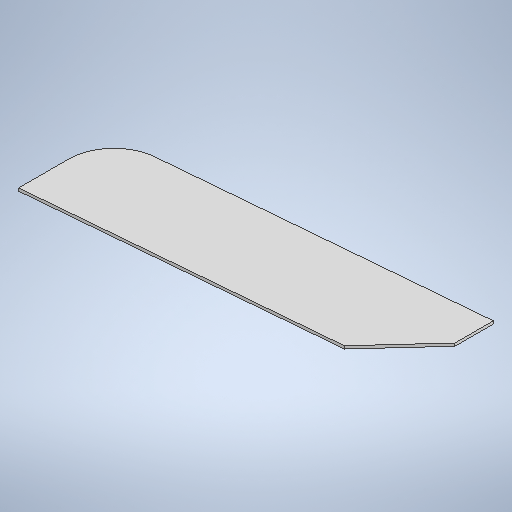
# Autodesk Inventor part: c
Saved by Autodesk Inventor 2025.2 (Build 292293000, 293)
## iProperties
Created: 2026-02-05
Part Number: c
Material: Generic
Document SubType Name: Modeling
Designer: Joefi
Density: 1 g/cm^3
Appearance: Default
Author: Joefi
Autodesk Inventor part; units mm, degrees
ref_plane "YZ Plane" through (0, 0, 0) normal (1, 0, 0) x (0, 1, 0)
ref_plane "XZ Plane" through (0, 0, 0) normal (0, 1, 0) x (-1, 0, 0)
ref_plane "XY Plane" through (0, 0, 0) normal (0, 0, 1) x (1, 0, 0)
sketch "Sketch1" plane through (0, 0, 0) normal (0, 1, 0) x (-1, 0, 0)
  line L0 (-55.6159, -9.9971) -> (-55.6159, -9.3981)
  arc A0 (-54.3022, -6.0201) -> (-55.6159, -9.3981) centre (-50.6159, -9.3981) ccw
  line L1 (-54.3022, -6.0201) -> (-42.899, 6.4243)
  arc A1 (-39.6484, 8.0273) -> (-42.899, 6.4243) centre (-39.2126, 3.0463) ccw
  line L2 (-39.6484, 8.0273) -> (35.5678, 14.6079)
  arc A2 (41.0036, 9.6269) -> (35.5678, 14.6079) centre (36.0036, 9.6269) ccw
  line L3 (41.0036, 9.6269) -> (41.0036, 3.0791)
  arc A3 (30.9623, -7.8791) -> (41.0036, 3.0791) centre (30.0036, 3.0791) ccw
  line L4 (30.9623, -7.8791) -> (-50.1801, -14.9781)
  arc A4 (-55.6159, -9.9971) -> (-50.1801, -14.9781) centre (-50.6159, -9.9971) ccw
  line L5 (-42.5345, 9.7825) -> (-57.6159, -6.6759)
  line L6 (-57.6159, -6.6759) -> (-57.6159, -17.6363)
  line L7 (-57.6159, -17.6363) -> (31.1366, -9.8715)
  arc A5 (31.1366, -9.8715) -> (43.0036, 3.0791) centre (30.0036, 3.0791) ccw
  line L8 (43.0036, 3.0791) -> (43.0036, 17.2661)
  line L9 (43.0036, 17.2661) -> (-42.5345, 9.7825)
  line L10 (-42.4396, 9.59) -> (-57.4159, -6.7537)
  line L11 (-57.4159, -6.7537) -> (-57.4159, -17.418)
  line L12 (-57.4159, -17.418) -> (31.1192, -9.6722)
  arc A6 (31.1192, -9.6722) -> (42.8036, 3.0791) centre (30.0036, 3.0791) ccw
  line L13 (42.8036, 3.0791) -> (42.8036, 17.0478)
  line L14 (42.8036, 17.0478) -> (-42.4396, 9.59)
  point P0 (0, 0)
  dimension "d0" = 0.2
  constraints: 30 end point, 14 point on circle, 7 centre point, 5 other
  measures "d0" distance between parallel lines of L9 L14
extrude "Extrusion1" add sketch "Sketch1" along normal blind 0.8 contours L0 A0 L1 A1 L2 A2 L3 A3 L4 A4 | L9 L8 A5 L7 L6 L5 | L14 L13 A6 L12 L11 L10
body "Solid1"
